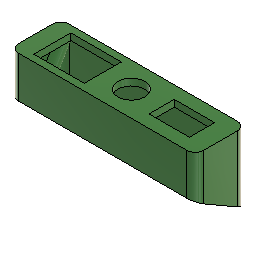
Power_button (Autodesk Fusion 360 design; units mm, degrees)
Autodesk Fusion 360 part; units mm, degrees
note: some values were not read from the file. Set by a fixed rule: which sketch regions a step uses.
sketch "Sketch1" plane through (0, 0, 0) normal (0, 0, 1) x (1, 0, 0)
  line L0 (-15, -11) -> (15, -11)
  line L1 (15, -11) -> (15, 11)
  line L2 (15, 11) -> (-15, 11)
  line L3 (-15, 11) -> (-15, -11)
  line L4 (-15, -11) -> (15, 11) construction
  line L5 (15, -11) -> (-15, 11) construction
  circle A0 centre (32, 0) radius 8
  line L6 (0, 0) -> (32, 0) construction
  line L7 (85, -15) -> (-25, -15)
  line L8 (-25, -15) -> (-25, 15)
  line L9 (-25, 15) -> (85, 15)
  line L10 (85, 15) -> (85, -15)
  line L11 (85, -15) -> (-25, 15) construction
  line L12 (-25, -15) -> (85, 15) construction
  line L13 (83, -13) -> (-23, -13)
  line L14 (-23, -13) -> (-23, 13)
  line L15 (-23, 13) -> (83, 13)
  line L16 (83, 13) -> (83, -13)
  line L17 (74, -7.5) -> (50, -7.5)
  line L18 (50, -7.5) -> (50, 7.5)
  line L19 (50, 7.5) -> (74, 7.5)
  line L20 (74, 7.5) -> (74, -7.5)
  line L21 (74, -7.5) -> (50, 7.5) construction
  line L22 (50, -7.5) -> (74, 7.5) construction
  line L23 (24, 13) -> (24, -13) construction
  line L24 (40, 13) -> (40, -13) construction
  line L25 (32, 0) -> (62, 0) construction
  point P0 (30, 0)
  point P1 (62, 0)
  dimension "d1" = 30
  dimension "d2" = 22
  dimension "d3" = 16
  dimension "d5" = 30
  dimension "d6" = 10
  dimension "d7" = 2
  dimension "d12" = 24
  dimension "d13" = 15
  dimension "d14" = 9
  dimension "d15" = 10
  dimension "d16" = 9
  dimension "d30" = 110
  constraint horizontal L0
  constraint perpendicular L0 L1
  constraint parallel L0 L2
  constraint parallel L1 L3
  constraint coincident L4 L6.start
  constraint coincident L5 L6.start
  constraint coincident L6.start origin
  constraint coincident A0.centre L6.end
  constraint horizontal L6
  constraint horizontal L7
  constraint perpendicular L7 L8
  constraint parallel L7 L9
  constraint parallel L8 L10
  constraint coincident L11 P0
  constraint coincident L12 P0
  constraint coincident L6 P0
  constraint horizontal L17
  constraint perpendicular L17 L18
  constraint parallel L17 L19
  constraint parallel L18 L20
  constraint coincident L21 P1
  constraint coincident L22 P1
  constraint coincident L15 L23.start
  constraint coincident L13 L23.end
  constraint perpendicular L13 L23
  constraint coincident L15 L24.start
  constraint coincident L13 L24.end
  constraint perpendicular L13 L24
  constraint tangent A0 L23
  constraint tangent A0 L24
  constraint coincident P1 L25.end
  constraint horizontal L25
  measures "d1" distance of L1.end L2.end
  measures "d2" distance of L0.end L1.end
  measures "d3" diameter of A0
  measures "d5" distance of L7.end L8.end
  measures "d6" horizontal distance of L2.end L8.end
  measures "d12" distance of L18.end L19.end
  measures "d13" distance of L17.end L18.end
  measures "d14" distance of L1 L23
  measures "d15" distance of L18 L24
  measures "d16" distance of L16 L20
  measures "d26" diameter of L9.end
  measures "d30" distance of L7.start L7.end
  measures "d32" diameter of L9.end
extrude "Extrude2" add sketch "Sketch1" against normal blind 4 contours L7 L8 L9 L10 | L13 L14 L15 L16 makes body 1
extrude "Extrude3" add sketch "Sketch1" against normal blind 42 contours L7 L8 L9 L10 bodies 1
extrude "Extrude4" add sketch "Sketch1" against normal blind 26.4 separate body contours L0 L1 L2 L3 makes body 2
sketch "Sketch4" plane through (-25, 0, 0) normal (-1, 0, 0) x (0, -1, 0)
  line L0 (15, 0) -> (-15, 0)
  line L1 (-15, 0) -> (-15, -42)
  line L2 (-15, -42) -> (15, -42)
  line L3 (15, -42) -> (15, 0)
  line L4 (-15, -42) -> (15, -24.6795)
  dimension "d24" = 60
  constraint coincident L1.end L2.start
  constraint coincident L3 L4.end
  measures "d24" angle of L1 L4
extrude "Extrude5" cut sketch "Sketch4" against normal through all contours L2 L3 L4 bodies 1 2
sketch "Sketch5" plane through (0, -14.4365, -25.0048) normal (0, -0.5, -0.866025) x (1, 0, 0)
  line L0 (-23, -1.6588) -> (83, -1.6588)
  line L1 (83, -1.6588) -> (83, -31.681)
  line L2 (83, -31.681) -> (-23, -31.681)
  line L3 (-23, -31.681) -> (-23, -1.6588)
  line L4 (85, -33.9904) -> (85, 0.6506)
  line L5 (85, 0.6506) -> (-25, 0.6506)
  line L6 (-25, 0.6506) -> (-25, -33.9904)
  line L7 (-25, -33.9904) -> (85, -33.9904)
  line L8 (-25, -11.5312) -> (85, -11.5312) construction
  circle A0 centre (-20, -11.5312) radius 1.5
  circle A1 centre (80, -11.5312) radius 1.5
  circle A2 centre (-20, -11.5312) radius 4
  circle A3 centre (80, -11.5312) radius 4
  line L9 (-25, -7.5312) -> (-20, -7.5312)
  line L10 (-25, -15.5312) -> (-20, -15.5312)
  line L11 (85, -7.5312) -> (80, -7.5312)
  line L12 (85, -15.5312) -> (80, -15.5312)
  dimension "d26" = 3
  dimension "d27" = 3
  dimension "d28" = 100
  dimension "d29" = 5
  dimension "d31" = 5
  dimension "d32" = 8
  dimension "d33" = 8
  constraint coincident L6 L8.start
  constraint coincident L4 L8.end
  constraint perpendicular L4 L8
  constraint coincident L8 A0.centre
  constraint coincident L8 A1.centre
  constraint concentric A0 A2
  constraint concentric A1 A3
  constraint coincident L6 L9.start
  constraint coincident A2 L9.end
  constraint tangent A2 L9
  constraint coincident L6 L10.start
  constraint coincident A2 L10.end
  constraint tangent A2 L10
  constraint horizontal L10
  constraint horizontal L9
  constraint coincident L4 L11.start
  constraint coincident A3 L11.end
  constraint tangent A3 L11
  constraint coincident L4 L12.start
  constraint coincident A3 L12.end
  constraint tangent A3 L12
  constraint horizontal L11
  constraint horizontal L12
  measures "d26" diameter of A0
  measures "d27" diameter of A1
  measures "d28" distance of A0.centre A1.centre
  measures "d29" distance of L8.start A0.centre
  measures "d31" distance of L8.end A1.centre
  measures "d32" diameter of A2
  measures "d33" diameter of A3
extrude "Extrude6" add sketch "Sketch5" against normal blind 31.9 contours L3 A2 L9 | L1 A3 L11 | L3 A2 | L1 A3 | L3 A2 L10 | L1 A3 L12 picked at (-22.5, -11.5312) picked at (82.5, -11.5312) bodies 1
fillet "Fillet3" radius 5 4 edges at (83, 13, -24.6955) (83, -13, -14.9171) (-23, 13, -24.6955) (-23, -13, -14.9171) on bodies 1
fillet "Fillet1" radius 2 2 edges at (30, -13, -4) (30, 13, -4) on bodies 1
sketch "Sketch6" plane through (0, 15, 0) normal (0, 1, 0) x (-1, 0, 0)
  line L0 (25, 0) -> (-85, 0)
  line L1 (-85, 0) -> (-85, -42)
  line L2 (-85, -42) -> (25, -42)
  line L3 (25, -42) -> (25, 0)
  circle A0 centre (-65, -42) radius 7.5
  circle A1 centre (-30, -42) radius 7.5
  circle A2 centre (5, -42) radius 7.5
  dimension "d39" = 15
  dimension "d40" = 15
  dimension "d41" = 15
  dimension "d42" = 20
  dimension "d43" = 20
  constraint coincident L2 A0.centre
  constraint midpoint L2 A1.centre
  constraint coincident L2 A2.centre
  measures "d39" diameter of A0
  measures "d40" diameter of A1
  measures "d41" diameter of A2
  measures "d42" distance of L1.end A0.centre
  measures "d43" distance of L2.end A2.centre
extrude "Extrude8" cut sketch "Sketch6" against normal blind 5 contours L2 A2 | L2 A0 | L2 A1 picked at (5.1868, -39.507) picked at (-65.5284, -39.1901) picked at (-29.8132, -39.507) bodies 1
fillet "Fillet2" radius 5 4 edges at (-25, -15, -12.3397) (-25, 15, -21) (85, -15, -12.3397) (85, 15, -21) on bodies 1
hidden bodies 2
named bodies: "Power_button"
